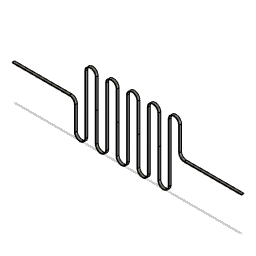
resistor (Autodesk Fusion 360 design; units mm, degrees)
Autodesk Fusion 360 part; units mm, degrees
note: some values were not read from the file. Set by a fixed rule: which sketch regions a step uses.
sketch "Sketch1" plane through (0, 0, 0) normal (0, 0, 1) x (1, 0, 0)
  line L0 (0, 0) -> (40, 0) construction
  arc A0 (10.9091, -0.9091) -> (10, 0) centre (10, -0.9091) ccw construction
  line L1 (10, -0.9091) -> (10.9091, -0.9091) construction
  line L2 (10.9091, -0.9091) -> (10.9091, -5.0909)
  arc A1 (10.9091, -5.0909) -> (12.7273, -5.0909) centre (11.8182, -5.0909) ccw
  line L3 (12.7273, -5.0909) -> (12.7273, 0)
  line L4 (11.8182, -6) -> (0, -6) construction
  line L5 (12.7273, 5.0909) -> (12.7273, 0)
  arc A2 (14.5455, 5.0909) -> (12.7273, 5.0909) centre (13.6364, 5.0909) ccw
  arc A3 (-29.3772, 59.3772) -> (30, 0) centre (30, 59.3772) ccw construction
  line L6 (-29.3772, 59.3772) -> (30, 59.3772) construction
  line L7 (14.5455, 5.0909) -> (14.5455, 0.9091)
  line L8 (30, 0) -> (40, 0)
  line L9 (10, 0) -> (0, 0)
  line L10 (13.6364, 6) -> (13.6364, 0) construction
  line L11 (10.9091, 0) -> (10.9091, -0.9091)
  arc A4 (14.5455, 0.9091) -> (15.4545, 0) centre (15.4545, 0.9091) ccw construction
  line L12 (14.5455, 0.9091) -> (14.5455, 0)
  line L13 (0, -0.05) -> (10, -0.05) construction
  arc A5 (10.8591, -0.9091) -> (10, -0.05) centre (10, -0.9091) ccw construction
  line L14 (10.8591, -0.9091) -> (10.8591, -5.0909)
  arc A6 (10.8591, -5.0909) -> (12.7773, -5.0909) centre (11.8182, -5.0909) ccw
  line L15 (12.7773, -5.0909) -> (12.7773, 5.0909)
  arc A7 (14.4955, 5.0909) -> (12.7773, 5.0909) centre (13.6364, 5.0909) ccw
  line L16 (14.4955, 5.0909) -> (14.4955, 0)
  line L17 (10.8591, -0.9091) -> (10.8591, 0)
  line L18 (0, 0.05) -> (10, 0.05) construction
  arc A8 (10.9591, -0.9091) -> (10, 0.05) centre (10, -0.9091) ccw construction
  line L19 (10.9591, -0.9091) -> (10.9591, -5.0909)
  arc A9 (10.9591, -5.0909) -> (12.6773, -5.0909) centre (11.8182, -5.0909) ccw
  line L20 (12.6773, -5.0909) -> (12.6773, 5.0909)
  arc A10 (14.5955, 5.0909) -> (12.6773, 5.0909) centre (13.6364, 5.0909) ccw
  line L21 (14.5955, 5.0909) -> (14.5955, 0)
  line L22 (0, 0.05) -> (0, -0.05)
  line L23 (10.9591, 0) -> (10.9591, -0.9091)
  arc A11 (-29.4272, 59.3772) -> (30, -0.05) centre (30, 59.3772) ccw construction
  line L24 (30, -0.05) -> (40, -0.05)
  arc A12 (-29.3272, 59.3772) -> (30, 0.05) centre (30, 59.3772) ccw construction
  line L25 (30, 0.05) -> (40, 0.05)
  line L26 (40, 0.05) -> (40, -0.05)
  line L27 (10.8591, 0) -> (10.9591, 0)
  line L28 (14.4955, 0) -> (14.5955, 0)
  point P0 (10, 0)
  point P1 (30, 0)
  dimension "d127" = 40
  dimension "d138" = 0.9091
  dimension "d142" = 6
  dimension "d148" = 360
  dimension "d151" = 10
  dimension "d152" = 10
  dimension "d161" = 6
  dimension "d162" = 1.8182
  dimension "d167" = 0.9091
  dimension "d177" = 0.05
  dimension "d182" = 0.05
  dimension "d187" = 0.05
  dimension "d188" = -0.05
  constraint coincident L0.start L9.end
  constraint tangent L0 A0
  constraint coincident P0 A0.end
  constraint coincident A0.centre L1.start
  constraint horizontal L1
  constraint tangent A0 L2
  constraint tangent L2 A1
  constraint coincident L0 L3.end
  constraint tangent A1 L3
  constraint perpendicular L0 L3
  constraint midpoint A1 L4.start
  constraint tangent A1 L4
  constraint horizontal L4
  constraint coincident L0 P1
  constraint coincident P1 A3.end
  constraint tangent L0 A3
  constraint coincident A3.centre L6.end
  constraint horizontal L6
  constraint coincident L0 P0
  constraint coincident L0 L12.end
  constraint tangent A2 L7
  constraint coincident L0 L11.start
  constraint midpoint A2 L10.start
  constraint coincident L0 L10.end
  constraint perpendicular L0 L10
  constraint vertical L11
  constraint tangent L0 A4
  constraint coincident L0 A4.end
  constraint tangent L7 A4
  constraint tangent A4 L12
  constraint parallel L1 L13
  constraint coincident L1 A5.start
  constraint tangent L13 A5
  constraint concentric A0 A5
  constraint tangent A5 L14
  constraint tangent L14 A6
  constraint concentric A1 A6
  constraint tangent A6 L15
  constraint vertical L15
  constraint tangent L15 A7
  constraint concentric A2 A7
  constraint coincident L0 L16.end
  constraint tangent A7 L16
  constraint perpendicular L0 L16
  constraint tangent A5 L17
  constraint coincident L0 L17.end
  constraint horizontal L18
  constraint tangent L18 A8
  constraint concentric A0 A8
  constraint vertical L19
  constraint tangent L19 A9
  constraint concentric A1 A9
  constraint tangent A9 L20
  constraint parallel L3 L20
  constraint tangent L20 A10
  constraint concentric A2 A10
  constraint coincident L0 L21.end
  constraint tangent A10 L21
  constraint coincident L0 L23.start
  constraint perpendicular L0 L23
  constraint coincident A8.start L19.start
  constraint vertical L26
  constraint tangent A8 L19
  constraint parallel L12 L21
  measures "d127" distance of L0.start L0.end
  measures "d138" radius of A0
  measures "d142" distance of L0.start L4
  measures "d151" distance of L0.start A0.end
  measures "d152" distance of L0.end P1
  measures "d161" vertical distance of L10.start L10.end
  measures "d162" distance of L5 L7
  measures "d167" radius of A4
  measures "d177" distance of L0 L13
  measures "d182" distance of L0 L18
extrude "Extrude3" add sketch "Sketch1" along normal blind 0.4 makes body 1
pattern_linear "R-Pattern1" count 5 spacing 3.6364 along (1, 0, 0) of bodies 1 makes body 2 at (16.4136, -1.697, 0.1333) makes body 3 at (20.05, -1.697, 0.1333) makes body 4 at (23.6864, -1.697, 0.1333) makes body 5 at (27.3227, -1.697, 0.1333)
sketch "Sketch3" plane through (0, 0, 0) normal (0, 0, 1) x (1, 0, 0)
  line L0 (0, 0) -> (10.9591, 0)
  line L1 (10.9591, 0) -> (10.9591, -0.9091)
  line L2 (10.9591, -0.9091) -> (0, -0.9091)
  line L3 (0, -0.9091) -> (0, 0)
  line L4 (40, 0) -> (29.0409, 0)
  line L5 (29.0409, 0) -> (29.0409, 0.9091)
  line L6 (29.0409, 0.9091) -> (40, 0.9091)
  line L7 (40, 0.9091) -> (40, 0)
  line L8 (0, 0) -> (40, 0)
  dimension "d199" = 10.9591
  dimension "d200" = 0.9091
  dimension "d201" = 40
  dimension "d202" = 29.0409
  dimension "d203" = 0.9091
  constraint horizontal L0
  constraint vertical L1
  constraint horizontal L2
  constraint vertical L3
  constraint coincident L0.start L3.end
  constraint horizontal L4
  constraint vertical L5
  constraint horizontal L6
  constraint vertical L7
  constraint collinear L4 L8
  measures "d199" distance of L1.end L2.end
  measures "d200" distance of L0.start L2.end
  measures "d201" horizontal distance of L0.start L4.start
  measures "d202" horizontal distance of L0.start L4.end
  measures "d203" distance of L4.start L6
extrude "Extrude4" cut sketch "Sketch3" along normal through all contours L0 L1 L2 L3 L8 bodies 1
sketch "Sketch6" plane through (0, 0, 0) normal (0, 0, 1) x (1, 0, 0)
  line L0 (29.0409, 0.9091) -> (40, 0.9091)
  line L1 (40, 0.9091) -> (40, 0)
  line L2 (40, 0) -> (29.0409, 0)
  line L3 (29.0409, 0) -> (29.0409, 0.9091)
  point P0 (40, 0.9091)
extrude "Extrude8" cut sketch "Sketch6" along normal blind 0.4 bodies 5
sketch "Sketch4" plane through (0, 0, 0) normal (0, 0, 1) x (1, 0, 0)
  line L0 (0, -0.05) -> (10, -0.05)
  arc A0 (10.8591, -0.9091) -> (10, -0.05) centre (10, -0.9091) ccw
  arc A1 (10.9591, -0.9091) -> (10, 0.05) centre (10, -0.9091) ccw
  line L1 (0, 0.05) -> (10, 0.05)
  line L2 (0, 0.05) -> (0, -0.05)
  line L3 (10.9591, -0.9091) -> (10.8591, -0.9091)
  line L4 (0, 0) -> (40, 0) construction
  point P0 (20, 0)
  dimension "d207" = 20
  dimension "d208" = 40
  constraint coincident L4.start origin
  constraint horizontal L4
  constraint coincident P0 L4
  measures "d207" horizontal distance of L4.start P0
  measures "d208" distance of L4.start L4.end
extrude "Extrude5" add sketch "Sketch4" along normal blind 0.4 separate body makes body 6
sketch "Sketch5" plane through (0, 0, 0) normal (0, 1, 0) x (1, 0, 0)
  line L0 (20, 5) -> (20, -5) construction
  point P0 (20, 0)
  dimension "d209" = 10
  dimension "d210" = 20
  constraint vertical L0
  constraint midpoint L0 P0
  measures "d209" distance of L0.start L0.end
  measures "d210" distance of L0 origin
pattern_circular "C-Pattern1" count 2 over 360 about axis through (20, 0, -5) along (0, 0, 1) of bodies 6 makes body 7
equation "d1000 = channelwidth"
equation "d4 = d1000 / 2"
equation "resistor_height = 12 mm"
equation "length = 40 mm"
equation "mouth_size = 2.2 * d1000" comment "Mouth size multiplier"
equation "channelwidth = 0.1 mm"
equation "depth = 0.4 mm"
equation "numcycles = 5"
equation "d127 = length"
equation "d138 = radius"
equation "radius = ( length - d151 * 2 ) / ( ( numcycles - 1 ) * 4 + 6 )"
equation "d142 = resistor_height / 2"
equation "d152 = d151"
equation "d161 = resistor_height / 2"
equation "d162 = radius * 2"
equation "d167 = radius"
equation "d177 = channelwidth / 2"
equation "d182 = channelwidth / 2"
equation "d187 = channelwidth / 2"
equation "d188 = -( channelwidth / 2 )"
equation "d193 = depth"
equation "d195 = numcycles"
equation "d197 = radius * 4"
equation "d199 = d151 + radius + channelwidth / 2"
equation "d200 = radius"
equation "d201 = length"
equation "d202 = length - d199"
equation "d203 = d200"
equation "d205 = depth"
equation "d207 = length / 2"
equation "d208 = length"
equation "d210 = length / 2"
equation "d216 = depth"
